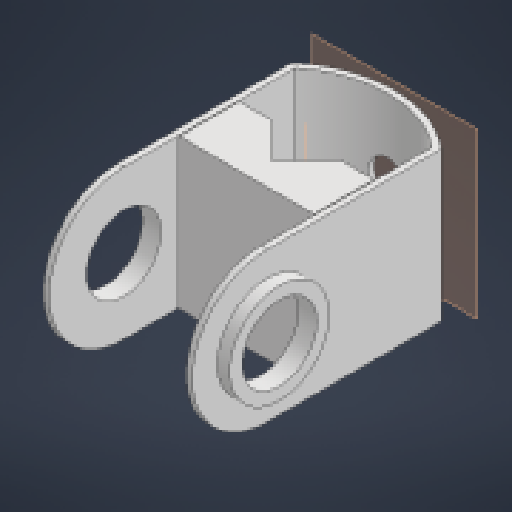
# Autodesk Inventor part: Clamp Body
Saved by Autodesk Inventor 2023.1 (Build 271208000, 208)
## iProperties
Created: 2022-12-06
Part Number: Clamp Body
Material: Generic
Document SubType Name: Modeling
Designer: aubrey-work
Density: 1 g/cm^3
Appearance: Default
Author: aubrey-work
Autodesk Inventor part; units mm, degrees
ref_plane "YZ Plane" through (0, 0, 0) normal (1, 0, 0) x (0, 1, 0)
ref_plane "XZ Plane" through (0, 0, 0) normal (0, 1, 0) x (-1, 0, 0)
ref_plane "XY Plane" through (0, 0, 0) normal (0, 0, 1) x (1, 0, 0)
sketch "Sketch1" plane through (0, 0, 0) normal (0, 1, 0) x (-1, 0, 0)
  line L0 (0, 0) -> (0, -63.5)
  arc A0 (0, -63.5) -> (38.1, -63.5) centre (19.05, -41.275) ccw
  line L1 (38.1, -63.5) -> (38.1, 0)
  line L2 (36.5125, 0) -> (36.5125, -62.7575)
  arc A1 (1.5875, -62.7574) -> (36.5125, -62.7575) centre (19.05, -41.275) ccw
  line L3 (1.5875, -62.7574) -> (1.5875, 0)
  line L4 (38.1, 0) -> (36.5125, 0)
  line L5 (1.5875, 0) -> (0, 0)
  circle A2 centre (19.05, -48.1951) radius 6.35 construction
  line L6 (12.7, -48.1951) -> (1.8415, -48.1951) construction
  line L7 (25.4, -48.1951) -> (36.2585, -48.1951) construction
  line L8 (19.05, -54.5451) -> (19.05, -68.9596) construction
  line L9 (12.7, -48.1951) -> (25.4, -48.1951) construction
  line L10 (10.0697, -48.1951) -> (19.05, -39.2148)
  line L11 (19.05, -39.2148) -> (28.0303, -48.1951)
  line L12 (28.0303, -48.1951) -> (36.2585, -48.1951)
  line L13 (10.0697, -48.1951) -> (1.8415, -48.1951)
  line L14 (1.8415, -32.8648) -> (36.2585, -32.8648)
  line L15 (1.8415, -48.1951) -> (1.8415, -32.8648)
  line L16 (36.2585, -48.1951) -> (36.2585, -32.8648)
  dimension "d0" = 63.5
  dimension "d1" = 38.1
  dimension "d2" = 38.1
  dimension "d3" = 1.5875
  dimension "d19" = 12.7
  dimension "d20" = 22.225
  dimension "d21" = 6.35
  dimension "d24" = 0.254
  dimension "d25" = 14.4145
  constraints: 34 end point, 8 point on circle, 4 perpendicular, 4 point on line, 3 centre point, 3 horizontal, 3 symmetric about line, 3 vertical, 2 equal length, 2 tangent, 1 collinear, 1 midpoint, 1 parallel, 2 other
  measures "d0" distance of L0.start L0.end
  measures "d1" distance of L0.end L1.start
  measures "d2" distance between parallel lines of L0 L1
  measures "d3" distance between parallel lines of L1 L2
  measures "d19" diameter of A2
  measures "d20" vertical distance of A0.centre L0.end
  measures "d21" distance from line of L14 L10.end
  measures "d24" distance from line of L3 L6.end
  measures "d25" distance of L8.start L8.end
extrude "Extrusion1" add sketch "Sketch1" along normal blind 38.1 contours L5 L3 A1 L2 L4 L1 A0 L0
ref_plane "Work Plane1" through (-19.05, 0, -70.5471) normal (0, 0, 1) x (1, 0, 0)
fillet "Fillet1" radius 19.05 4 edges at (-0.7937, 38.1, 0) (-37.3062, 38.1, 0) (-37.3062, 0, 0) (-0.7937, 0, 0)
sketch "Sketch2" plane through (0, 0, -63.5) normal (1, 0, 0) x (0, 0, -1)
  arc A0 (-44.45, 38.1) -> (-44.45, 0) centre (-44.45, 19.05) ccw projected
  line L0 (-44.45, 0) -> (0, 0) projected
  line L1 (0, 0) -> (0, 38.1) projected
  line L2 (-44.45, 38.1) -> (0, 38.1) projected
  circle A1 centre (-44.45, 19.05) radius 9.525
  circle A2 centre (-44.45, 19.05) radius 12.7
  point P0 (-63.5, 0)
  dimension "d7" = 19.05
  dimension "d8" = 3.175
  constraints: 2 centre point, 1 coincident
  measures "d7" diameter of A1
  measures "d8" radial gap between concentric circles of A1 A2
extrude "Extrusion2" cut sketch "Sketch2" against normal through all contours A1
extrude "Extrusion3" add sketch "Sketch2" along normal blind 3.175 contours A2
extrude "Extrusion4" add sketch "Sketch2" against normal blind 3.175 from surface at -38.1 contours A2
sketch "Sketch3" plane through (-19.05, 0, -70.5471) normal (0, 0, 1) x (1, 0, 0)
  line L0 (19.05, 0) -> (-19.05, 0) projected
  line L1 (-19.05, 0) -> (-19.05, 38.1) projected
  line L2 (19.05, 38.1) -> (-19.05, 38.1) projected
  line L3 (19.05, 0) -> (19.05, 38.1) projected
  line L4 (19.05, 38.1) -> (-19.05, 0) construction
  circle A0 centre (0, 19.05) radius 4.7625
  point P0 (19.05, 0)
  dimension "d6" = 19.05
  dimension "d15" = 9.525
  constraints: 2 end point, 1 centre point, 1 midpoint
  measures "d15" diameter of A0
extrude "screw hole" cut sketch "Sketch3" along normal through all contours A0
extrude "Extrusion6" add sketch "Sketch1" along normal up to surface (38.1 mm away) contours L13 L15 L14 L16 L12 L11 L10
body "Solid1"
